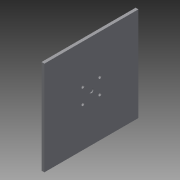
# Autodesk Inventor part: marker plate
Saved by Autodesk Inventor 2014 (Build 180170000, 170)
## iProperties
Created: 2014-11-30
Part Number: marker plate
Material: Generic
Document SubType Name: Modeling
Designer: ph1140784
Density: 1 g/cm^3
Appearance: Default
Mass: 29.8996 g
Surface Area: 212.705 cm^2
Volume: 29.8996 cm^3
Author: ph1140784
Autodesk Inventor part; units mm, degrees
ref_plane "YZ Plane" through (0, 0, 0) normal (1, 0, 0) x (0, 1, 0)
ref_plane "XZ Plane" through (0, 0, 0) normal (0, 1, 0) x (-1, 0, 0)
ref_plane "XY Plane" through (0, 0, 0) normal (0, 0, 1) x (1, 0, 0)
sketch "Sketch1" plane through (0, 0, 0) normal (1, 0, 0) x (0, 1, 0)
  line L0 (50, 50) -> (-50, 50)
  line L1 (-50, 50) -> (-50, -50)
  line L2 (-50, -50) -> (50, -50)
  line L3 (50, -50) -> (50, 50)
  line L4 (50, 50) -> (-50, -50) construction
  line L5 (-50, 50) -> (50, -50) construction
  point P0 (0, 0)
  dimension "d0" = 100
  dimension "d1" = 100
  constraints: 12 end point, 2 midpoint, 2 parallel, 1 horizontal, 1 perpendicular
  measures "d0" distance of L2.end L1.end
  measures "d1" distance of L1.end L0.end
extrude "Extrusion1" add sketch "Sketch1" along normal blind 3
sketch "Sketch2" plane through (3, 0, 0) normal (1, 0, 0) x (0, 0, -1)
  circle A0 centre (-8, -9) radius 1.5
  circle A1 centre (8, -9) radius 1.5
  circle A2 centre (8, 9) radius 1.5
  circle A3 centre (-8, 9) radius 1.5
  ellipse E0 centre (0, 0) end of major axis (13, 14) minor radius 3.6924 (4.9841, 0.0284) -> (0.0262, 5.3386) ccw
  ellipse E1 centre (0, 0) end of major axis (-13, 14) minor radius 3.7302 (0.0262, 5.3386) -> (-4.9841, -0.0284) ccw
  ellipse E2 centre (0, 0) end of major axis (13, 14) minor radius 3.6924 (-4.9841, -0.0284) -> (-0.0262, -5.3386) ccw
  ellipse E3 centre (0, 0) end of major axis (-13, 14) minor radius 3.7302 (-0.0262, -5.3386) -> (4.9841, 0.0284) ccw
  point P0 (0, 9.3923)
  constraints: 4 centre point, 16 other
extrude "Extrusion2" cut sketch "Sketch2" against normal blind 3 contours A0 | A1 | A2 | A3
sketch "Sketch3" plane through (3, 0, 0) normal (1, 0, 0) x (0, 0, -1)
  circle A0 centre (0, 0) radius 2.2245
  constraints: 1 centre point, 1 coincident
extrude "Extrusion3" cut sketch "Sketch3" against normal blind 1
body "Solid1"
